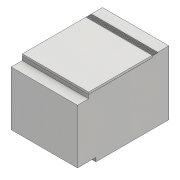
# Autodesk Inventor part: mieleWT946
Saved by Autodesk Inventor 2018 (Build 220112000, 112)
## iProperties
Created: 2017-12-11
Part Number: mieleWT946
Material: ABS Plastic
Document SubType Name: Modeling
Designer: sawaiz
Density: 1.06 g/cm^3
Appearance: Paint
Author: sawaiz
Autodesk Inventor part; units mm, degrees
ref_plane "YZ Plane" through (0, 0, 0) normal (1, 0, 0) x (0, 1, 0)
ref_plane "XZ Plane" through (0, 0, 0) normal (0, 1, 0) x (-1, 0, 0)
ref_plane "XY Plane" through (0, 0, 0) normal (0, 0, 1) x (1, 0, 0)
sketch "Sketch1" plane through (0, 0, 0) normal (0, 1, 0) x (-1, 0, 0)
  line L0 (297.5, 287.5) -> (-297.5, 287.5)
  line L1 (-297.5, 287.5) -> (-297.5, -287.5)
  line L2 (-297.5, -287.5) -> (297.5, -287.5)
  line L3 (297.5, -287.5) -> (297.5, 287.5)
  line L4 (297.5, 287.5) -> (-297.5, -287.5) construction
  line L5 (-297.5, 287.5) -> (297.5, -287.5) construction
  point P0 (0, 0)
  dimension "d0" = 595
  dimension "d1" = 575
  constraints: 12 end point, 2 midpoint, 2 parallel, 1 horizontal, 1 perpendicular
  measures "d0" distance of L2.end L1.end
  measures "d1" distance of L1.end L0.end
extrude "Extrusion1" add sketch "Sketch1" along normal blind 820
sketch "Sketch2" plane through (297.5, 0, 287.5) normal (1, 0, 0) x (0, 0, -1)
  line L0 (0, 0) -> (575, 0) projected
  line L1 (575, 0) -> (575, 820) projected
  line L2 (0, 820) -> (575, 820) projected
  line L3 (0, 0) -> (0, 820) projected
  line L4 (0, 0) -> (575, 0) projected
  line L5 (575, 0) -> (540, 0)
  line L6 (540, 0) -> (540, 165)
  line L7 (540, 165) -> (575, 165)
  line L8 (575, 165) -> (575, 0)
  point P0 (287.5, 0)
  dimension "d4" = 35
  dimension "d5" = 165
  constraints: 8 end point, 2 parallel, 1 horizontal, 1 perpendicular
  measures "d4" distance of L6.end L7.end
  measures "d5" distance of L5.end L6.end
extrude "Extrusion2" cut sketch "Sketch2" against normal through all contours L6 L7 L1 L0
sketch "Sketch3" plane through (297.5, 0, 287.5) normal (1, 0, 0) x (0, 0, -1)
  line L0 (540, 0) -> (540, 165) projected
  line L1 (540, 165) -> (575, 165) projected
  line L2 (575, 165) -> (575, 820) projected
  line L3 (0, 820) -> (575, 820) projected
  line L4 (0, 0) -> (0, 820) projected
  line L5 (0, 0) -> (540, 0) projected
  line L6 (0, 0) -> (52, 0)
  line L7 (52, 0) -> (52, 100)
  line L8 (52, 100) -> (0, 100)
  line L9 (0, 100) -> (0, 0)
  point P0 (287.5, 0)
  dimension "d8" = 52
  dimension "d9" = 100
  constraints: 8 end point, 2 parallel, 1 horizontal, 1 perpendicular
  measures "d8" distance of L8.end L7.end
  measures "d9" distance of L7.end L6.end
extrude "Extrusion3" cut sketch "Sketch3" against normal through all contours L5 L4 L8 L7
sketch "Sketch4" plane through (-297.5, 820, 287.5) normal (0, 0, 1) x (1, 0, 0)
  line L0 (0, -720) -> (595, -720) projected
  line L1 (595, -720) -> (595, 0) projected
  line L2 (0, 0) -> (595, 0) projected
  line L3 (0, -720) -> (0, 0) projected
  line L4 (595, -720) -> (595, 0) projected
  line L5 (0, -720) -> (595, -720)
  line L6 (595, -720) -> (595, -150)
  line L7 (595, -150) -> (0, -150)
  line L8 (0, -150) -> (0, -720)
  point P0 (297.5, -820)
  dimension "d12" = 570
  constraints: 8 end point, 2 parallel, 1 horizontal, 1 perpendicular, 1 point on line
  measures "d12" distance of L6.end L5.end
extrude "Extrusion4" cut sketch "Sketch4" against normal blind 19 contours L3 L7 L1 L0
sketch "Sketch5" plane through (-297.5, 820, 268.5) normal (0, 0, 1) x (1, 0, 0)
  line L0 (595, -720) -> (0, -720) projected
  line L1 (595, -150) -> (595, -720) projected
  line L2 (0, -150) -> (595, -150) projected
  line L3 (0, -720) -> (0, -150) projected
  line L4 (0.5, -720) -> (594.5, -720)
  line L5 (594.5, -720) -> (594.5, -150)
  line L6 (594.5, -150) -> (0.5, -150)
  line L7 (0.5, -150) -> (0.5, -720)
  point P0 (297.5, -820)
  dimension "d15" = 0.5
  dimension "d16" = 0.5
  constraints: 8 end point, 2 parallel, 2 point on line, 1 horizontal, 1 perpendicular
  measures "d15" distance between parallel lines of L1 L5
  measures "d16" distance between parallel lines of L3 L7
extrude "Extrusion5" add sketch "Sketch5" along normal blind 19 separate body contours L0 L7 L2 L5
sketch "Sketch6" plane through (-297.5, 820, 287.5) normal (0, 0, 1) x (1, 0, 0)
  line L0 (0, -150) -> (595, -150) projected
  line L1 (595, -150) -> (595, 0) projected
  line L2 (0, 0) -> (595, 0) projected
  line L3 (0, -150) -> (0, 0) projected
  line L4 (595, -145) -> (0, -145)
  line L5 (0, -145) -> (0, -140)
  line L6 (0, -140) -> (595, -140)
  line L7 (595, -140) -> (595, -145)
  point P0 (297.5, -820)
  dimension "d19" = 5
  dimension "d20" = 5
  constraints: 8 end point, 2 parallel, 2 point on line, 1 horizontal, 1 perpendicular
  measures "d19" distance between parallel lines of L4 L0
  measures "d20" distance between parallel lines of L6 L4
extrude "Extrusion6" cut sketch "Sketch6" against normal blind 5 contours L3 L6 L1 L4 bodies 1
pattern_linear "Rectangular Pattern1" count 5 spacing 10 along (0, 1, 0) of "Extrusion6" bodies 1
body "Solid1"
body "Solid2"
